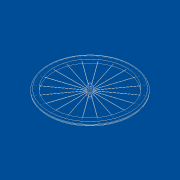
# Autodesk Inventor part: Rueda
Saved by Autodesk Inventor 2016 (Build 200138000, 138)
## iProperties
Created: 2017-05-13
Part Number: Rueda
Material: Generic
Document SubType Name: Modeling
Designer: Gian
Density: 1 g/cm^3
Appearance: Default
Author: Gian
Autodesk Inventor part; units mm, degrees
ref_plane "YZ Plane" through (0, 0, 0) normal (1, 0, 0) x (0, 1, 0)
ref_plane "XZ Plane" through (0, 0, 0) normal (0, 1, 0) x (-1, 0, 0)
ref_plane "XY Plane" through (0, 0, 0) normal (0, 0, 1) x (1, 0, 0)
sketch "Sketch1" plane through (0, 0, 0) normal (0, 0, 1) x (1, 0, 0)
  circle A0 centre (0, 0) radius 298.5
  circle A1 centre (0, 0) radius 255.8492
  circle A2 centre (0, 0) radius 7.5
  circle A3 centre (0, 0) radius 11.5295
  circle A4 centre (0, 0) radius 18.1436
  circle A5 centre (0, 0) radius 22.8175
  circle A6 centre (0, 0) radius 7
  dimension "d0" = 597
  dimension "d1" = 15
  dimension "d9" = 14
  constraints: 7 centre point, 5 coincident
  measures "d0" diameter of A0
  measures "d1" diameter of A2
  measures "d9" diameter of A6
extrude "Extrusion1" add sketch "Sketch1" along normal mid plane 25 contours A0
fillet "Fillet1" radius 10 2 edges at (-298.5, 0, 12.5) (-298.5, 0, -12.5)
extrude "Extrusion2" add sketch "Sketch1" along normal mid plane 62 contours A3
extrude "Extrusion3" add sketch "Sketch1" along normal mid plane 50 contours A4
extrude "Extrusion4" add sketch "Sketch1" along normal mid plane 90 contours A6
sketch "Sketch2" plane through (0, 0, 0) normal (1, 0, 0) x (0, 1, 0)
  circle A0 centre (0, 0) radius 0.7678
  line L0 (7, 45) -> (-7, 45) projected
  line L1 (-7, -45) -> (7, -45) projected
  line L2 (0, 45) -> (0, -45)
  constraints: 4 midpoint, 2 end point, 1 centre point
extrude "Extrusion5" add sketch "Sketch2" along normal blind 280 separate body
pattern_circular "Circular Pattern1" count 20 over 360 about axis through (0, 0, 45) along (0, 0, 1) of "Extrusion5" bodies 2
body "Solid1"
body "Solid2"
